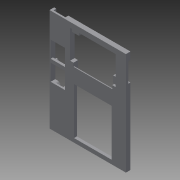
# Autodesk Inventor part: DisplayTop
Saved by Autodesk Inventor 2014 SP1 (Build 180222100, 222)
## iProperties
Created: 2014-03-24
Part Number: DisplayTop
Material: Generic
Document SubType Name: Modeling
Designer: patrigg
Density: 1 g/cm^3
Appearance: Default
Author: patrigg
Autodesk Inventor part; units mm, degrees
ref_plane "YZ Plane" through (0, 0, 0) normal (1, 0, 0) x (0, 1, 0)
ref_plane "XZ Plane" through (0, 0, 0) normal (0, 1, 0) x (-1, 0, 0)
ref_plane "XY Plane" through (0, 0, 0) normal (0, 0, 1) x (1, 0, 0)
sketch "Sketch2" plane through (0, 0, 0) normal (0, 1, 0) x (-1, 0, 0)
  line L0 (-33.5, -45) -> (33.5, -45)
  line L1 (33.5, -45) -> (33.5, 45)
  line L2 (33.5, 45) -> (-33.5, 45)
  line L3 (-33.5, 45) -> (-33.5, -45)
  line L4 (-33.5, -45) -> (33.5, 45) construction
  line L5 (33.5, -45) -> (-33.5, 45) construction
  point P0 (0, 0)
  dimension "d0" = 67
  dimension "d1" = 90
  constraints: 12 end point, 2 midpoint, 2 parallel, 1 horizontal, 1 perpendicular
  measures "d0" distance of L2.end L1.end
  measures "d1" distance of L1.end L0.end
extrude "Extrusion1" add sketch "Sketch2" along normal blind 4
sketch "Sketch3" plane through (0, 4, 0) normal (0, 1, 0) x (1, 0, 0)
  line L0 (33.5, 45) -> (-33.5, 45) projected
  line L1 (-14.5, -9.5) -> (23.5, -9.5)
  line L2 (23.5, -9.5) -> (23.5, 43)
  line L3 (23.5, 43) -> (-14.5, 43)
  line L4 (-14.5, 43) -> (-14.5, -9.5)
  line L5 (-14.5, -9.5) -> (23.5, 43) construction
  line L6 (23.5, -9.5) -> (-14.5, 43) construction
  line L7 (33.5, -45) -> (33.5, 45) projected
  point P0 (0, 0)
  point P1 (4.5, 16.75)
  dimension "d4" = 38
  dimension "d5" = 52.5
  dimension "d6" = 2
  dimension "d99" = 10
  constraints: 12 end point, 2 midpoint, 2 parallel, 1 horizontal, 1 perpendicular
  measures "d4" distance of L3.end L2.end
  measures "d5" distance of L2.end L1.end
  measures "d6" distance between parallel lines of L0 L3
  measures "d99" distance between parallel lines of L7 L2
extrude "Extrusion2" cut sketch "Sketch3" against normal blind 1.5
sketch "Sketch4" plane through (0, 2.5, 0) normal (0, 1, 0) x (1, 0, 0)
  line L0 (23.5, -9.5) -> (-14.5, -9.5) projected
  line L1 (23.5, 43) -> (23.5, -9.5) projected
  line L2 (-14.5, 43) -> (23.5, 43) projected
  line L3 (-14.5, -9.5) -> (-14.5, 43) projected
  line L4 (-12, 41.5) -> (21, 41.5)
  line L5 (21, 41.5) -> (21, 0.5)
  line L6 (21, 0.5) -> (-12, 0.5)
  line L7 (-12, 0.5) -> (-12, 41.5)
  line L8 (-12, 41.5) -> (21, 0.5) construction
  line L9 (21, 41.5) -> (-12, 0.5) construction
  point P0 (0, 0)
  point P1 (4.5, 21)
  dimension "d9" = 10
  dimension "d10" = 1.5
  dimension "d11" = 2.5
  dimension "d12" = 2.5
  constraints: 12 end point, 2 midpoint, 2 parallel, 1 horizontal, 1 perpendicular
  measures "d9" distance between parallel lines of L0 L6
  measures "d10" distance between parallel lines of L2 L4
  measures "d11" distance between parallel lines of L1 L5
  measures "d12" distance between parallel lines of L3 L7
extrude "Extrusion3" cut sketch "Sketch4" against normal blind 2.5 contours L4 L5 L6 L7
sketch "Sketch5" plane through (0, 4, 0) normal (0, 1, 0) x (1, 0, 0)
  line L0 (23.5, 43) -> (23.5, -9.5) projected
  line L1 (23.5, -9.5) -> (-14.5, -9.5) projected
  line L2 (-14.5, -9.5) -> (-14.5, 43) projected
  line L3 (-12.5, -15.5) -> (-12.5, -9.5)
  line L4 (21.5, -15.5) -> (21.5, -9.5)
  line L5 (33.5, 45) -> (-33.5, 45) projected
  line L6 (-12.5, -15.5) -> (21.5, -15.5)
  point P0 (0, 0)
  dimension "d18" = 2
  dimension "d19" = 2
  constraints: 6 end point, 2 perpendicular, 2 point on line, 1 parallel
  measures "d18" distance between parallel lines of L3 L2
  measures "d19" distance between parallel lines of L0 L4
extrude "Extrusion4" cut sketch "Sketch5" against normal blind 0.25
sketch "Sketch12" plane through (0, 4, 0) normal (0, 1, 0) x (1, 0, 0)
  line L0 (21.5, -15.5) -> (-12.5, -15.5) projected
  line L1 (-15.5, -40.5) -> (24.5, -40.5)
  line L2 (24.5, -40.5) -> (24.5, -15.5)
  line L3 (24.5, -15.5) -> (-15.5, -15.5)
  line L4 (-15.5, -15.5) -> (-15.5, -40.5)
  line L5 (-15.5, -40.5) -> (24.5, -15.5) construction
  line L6 (24.5, -40.5) -> (-15.5, -15.5) construction
  line L7 (23.5, 43) -> (23.5, -9.5) projected
  point P0 (0, 0)
  point P1 (4.5, -28)
  point P2 (4.5, -28)
  dimension "d58" = 40
  dimension "d59" = 25
  dimension "d100" = 1
  constraints: 12 end point, 3 midpoint, 2 parallel, 1 collinear, 1 horizontal, 1 perpendicular
  measures "d58" distance of L3.end L2.end
  measures "d59" distance of L2.end L1.end
  measures "d100" distance between parallel lines of L2 L7
extrude "Extrusion10" cut sketch "Sketch12" against normal blind 4
sketch "Sketch13" plane through (24.5, 4, 15.5) normal (-1, 0, 0) x (0, 0, 1)
  line L0 (0, 0) -> (25, 0) projected
  line L1 (0, 0) -> (0, -4) projected
  line L2 (25, -4) -> (0, -4) projected
  line L3 (6, 0) -> (6, -4)
  line L4 (0, -2.2) -> (6, -2.2)
  point P0 (-15.5, -4)
  dimension "d67" = 6
  dimension "d74" = 1.8
  constraints: 4 end point, 4 point on line, 2 perpendicular
  measures "d67" distance between parallel lines of L3 L1
  measures "d74" distance between parallel lines of L2 L4
sketch "Sketch14" plane through (-15.5, 4, 40.5) normal (1, 0, 0) x (0, 0, -1)
  line L0 (0, 0) -> (25, 0) projected
  line L1 (0, 0) -> (0, -4)
  line L2 (4.0418, -2.2) -> (4.0418, 0)
  line L3 (25, -4) -> (0, -4) projected
  line L4 (0, -2.2) -> (4.0418, -2.2)
  point P0 (40.5, -4)
  point P1 (0, -2)
  dimension "d79" = 1.8
  constraints: 6 end point, 2 perpendicular, 2 point on line, 1 midpoint
  measures "d79" distance between parallel lines of L3 L4
extrude "Extrusion13" add sketch "Sketch13" along normal blind 4 contours L0 L3 L4 L1
extrude "Extrusion14" add sketch "Sketch14" along normal blind 6
sketch "Sketch16" plane through (0, 3.75, 0) normal (0, 1, 0) x (1, 0, 0)
  line L0 (-12.5, -15.5) -> (-12.5, -9.5) projected
  line L1 (20.5, -15.5) -> (-12.5, -15.5) projected
  line L2 (21.5, -15.5) -> (20.5, -15.5) projected
  line L3 (21.5, -9.5) -> (21.5, -15.5) projected
  line L4 (-12.5, -9.5) -> (21.5, -9.5) projected
  point P0 (0, 0)
extrude "Extrusion15" cut sketch "Sketch16" against normal up to next
sketch "Sketch17" plane through (21.5, 4, 9.5) normal (-1, 0, 0) x (0, 0, 1)
  line L0 (0, -1.5) -> (0, -4) projected
  line L1 (6, -4) -> (0, -4) projected
  line L2 (6, -2.2) -> (6, -4) projected
  line L3 (6, 0) -> (6, -2.2) projected
  line L4 (0, -1.5) -> (-1.7339, -1.5) construction
  line L5 (5, -4) -> (7.1842, -4) construction
  line L6 (0, -1.5) -> (5, -4) construction
  arc A0 (2.5, -2.75) -> (0, -1.5) centre (0, -4.625) ccw
  line L7 (0, -1.5) -> (0, 0) projected
  line L8 (2.5, -2.75) -> (3.4375, -4)
  line L9 (2.9125, -4) -> (2.9125, -3.3)
  point P0 (-9.5, -4)
  dimension "d82" = 1
  dimension "d86" = 0.7
  constraints: 10 end point, 4 point on line, 2 parallel, 2 point on circle, 2 tangent, 1 centre point, 1 midpoint, 1 perpendicular
  measures "d82" distance from line of L2 L5.start
  measures "d86" distance of L9.start L9.end
extrude "Extrusion16" add sketch "Sketch17" along normal up to next contours A0 L8 L9 L1 L0
fillet "Fillet5" radius 1 1 edges at (4.5, 0.7, 12.4125)
sketch "Sketch18" plane through (0, 4, 0) normal (0, 1, 0) x (1, 0, 0)
  line L0 (-33.5, 45) -> (-33.5, -45) projected
  line L1 (-32.5, 9) -> (-20, 9)
  line L2 (-20, 9) -> (-20, -23)
  line L3 (-20, -23) -> (-32.5, -23)
  line L4 (-32.5, -23) -> (-32.5, 9)
  line L5 (33.5, 45) -> (-33.5, 45) projected
  point P0 (0, 0)
  dimension "d89" = 1
  dimension "d97" = 12.5
  dimension "d98" = 32
  dimension "d157" = 36
  constraints: 8 end point, 2 parallel, 1 horizontal, 1 perpendicular
  measures "d89" distance between parallel lines of L0 L4
  measures "d97" distance between parallel lines of L2 L4
  measures "d98" distance between parallel lines of L1 L3
  measures "d157" distance between parallel lines of L1 L5
extrude "Extrusion17" cut sketch "Sketch18" against normal up to next
sketch "Sketch19" plane through (-32.5, 4, 23) normal (1, 0, 0) x (0, 0, -1)
  line L0 (32, -4) -> (0, -4) projected
  line L1 (0, 0) -> (0, -4) projected
  line L2 (14.5, -4) -> (17.5, -4)
  line L3 (17.5, -4) -> (17.5, -2)
  line L4 (17.5, -2) -> (14.5, -2)
  line L5 (14.5, -2) -> (14.5, -4)
  line L6 (14.5, -4) -> (17.5, -2) construction
  line L7 (17.5, -4) -> (14.5, -2) construction
  point P0 (16, -3)
  dimension "d106" = 3
  dimension "d107" = 2
  dimension "d108" = 16
  constraints: 12 end point, 2 midpoint, 2 parallel, 1 collinear, 1 horizontal, 1 perpendicular
  measures "d106" distance of L4.end L3.end
  measures "d107" distance of L3.end L2.end
  measures "d108" distance from line of L1 point (16, -3)
extrude "Extrusion18" add sketch "Sketch19" along normal up to next
sketch "Sketch21" plane through (-32.5, 2, 8.5) normal (0, 1, 0) x (1, 0, 0)
  line L0 (0, 3) -> (12.5, 3) projected
  line L1 (0, 0) -> (12.5, 0) projected
  line L2 (4.75, 1) -> (7.75, 1)
  line L3 (7.75, 1) -> (7.75, 3)
  line L4 (7.75, 3) -> (4.75, 3)
  line L5 (4.75, 3) -> (4.75, 1)
  line L6 (4.75, 1) -> (7.75, 3) construction
  line L7 (7.75, 1) -> (4.75, 3) construction
  point P0 (32.5, 8.5)
  point P1 (6.25, 2)
  point P2 (6.25, 2)
  point P3 (6.25, 0)
  dimension "d111" = 3
  dimension "d112" = 2
  constraints: 12 end point, 4 midpoint, 2 parallel, 1 collinear, 1 horizontal, 1 perpendicular, 1 vertical alignment
  measures "d111" distance of L4.end L3.end
  measures "d112" distance of L3.end L2.end
extrude "Extrusion19" cut sketch "Sketch21" against normal blind 0.5
fillet "Fillet6" radius 1 1 edges at (-26.25, 1.5, 5.5)
sketch "Sketch22" plane through (-32.5, 2, 8.5) normal (0, 1, 0) x (1, 0, 0)
  line L0 (0, 0) -> (12.5, 0) projected
  line L1 (12.5, 3) -> (12.5, 0) projected
  circle A0 centre (2.125, 1.5) radius 1.25
  circle A1 centre (10.375, 1.5) radius 1.25
  point P0 (32.5, 8.5)
  point P1 (6.25, 1.5)
  point P2 (6.25, 0)
  point P3 (12.5, 1.5)
  dimension "d116" = 2.5
  dimension "d117" = 2.5
  dimension "d118" = 8.25
  dimension "d119" = 4.125
  constraints: 3 horizontal alignment, 2 centre point, 2 midpoint, 1 vertical alignment
  measures "d116" diameter of A0
  measures "d117" diameter of A1
  measures "d118" distance of A1.centre A0.centre
  measures "d119" distance of A0.centre point (6.25, 1.5)
extrude "Extrusion20" add sketch "Sketch22" along normal blind 2
chamfer "Chamfer3" distance 0.5 angle 45 2 edges at (-31.625, 4, 7) (-23.375, 4, 7)
sketch "Sketch23" plane through (0, 4, 0) normal (0, 1, 0) x (1, 0, 0)
  line L0 (-33.5, 45) -> (-33.5, -45) projected
  line L1 (-33.5, -45) -> (33.5, -45) projected
  line L2 (-31.5, -29) -> (-21, -29)
  line L3 (-21, -29) -> (-21, -45)
  line L4 (-21, -45) -> (-31.5, -45)
  line L5 (-31.5, -45) -> (-31.5, -29)
  line L6 (-31.5, -29) -> (-21, -45) construction
  line L7 (-21, -29) -> (-31.5, -45) construction
  line L8 (21.5, -9.5) -> (21.5, -15.5) projected
  line L9 (-31.25, -29) -> (-31.25, -37)
  line L10 (-31.25, -37) -> (-31.5, -37)
  line L11 (-21.25, -29) -> (-21.25, -37)
  line L12 (-21.25, -37) -> (-21, -37)
  point P0 (0, 0)
  point P1 (-26.25, -37)
  dimension "d125" = 10.5
  dimension "d126" = 16
  dimension "d127" = 7.25
  dimension "d130" = 0.25
  dimension "d131" = 0.25
  dimension "d132" = 8
  constraints: 20 end point, 4 midpoint, 4 perpendicular, 3 parallel, 2 collinear, 2 point on line, 1 horizontal
  measures "d125" distance of L3.end L4.end
  measures "d126" distance of L2.end L3.end
  measures "d127" distance from line of L0 point (-26.25, -37)
  measures "d130" distance between parallel lines of L5 L9
  measures "d131" distance between parallel lines of L3 L11
  measures "d132" distance of L4.end L10.end
extrude "Extrusion22" cut sketch "Sketch23" against normal blind 2.5 contours L5 L10 L9 L2 L11 L12 L3 L1
sketch "Sketch24" plane through (0, 4, 0) normal (0, 1, 0) x (1, 0, 0)
  line L0 (21.5, -15.5) -> (20.5, -15.5) projected
  line L1 (-31.25, -37) -> (-31.25, -29) projected
  line L2 (-31.25, -29) -> (-21.25, -29) projected
  line L3 (-21.25, -29) -> (-21.25, -37) projected
  line L4 (-32.5, 9) -> (-20, 9) projected
  line L5 (-20, 9) -> (-20, -23) projected
  line L6 (-20, -23) -> (-32.5, -23) projected
  line L7 (-27.5, 9) -> (-27.5, 17.5)
  line L8 (-27.5, 17.5) -> (-16.5, 17.5)
  line L9 (-16.5, 17.5) -> (-16.5, -29)
  line L10 (-16.5, -29) -> (-21.25, -29)
  line L11 (-25, 9) -> (-25, 15)
  line L12 (-25, 15) -> (-19, 15)
  line L13 (-19, 15) -> (-19, -25)
  line L14 (-19, -25) -> (-28.25, -25)
  line L15 (-28.25, -25) -> (-28.25, -29)
  point P0 (0, 0)
  point P1 (-26.25, 9)
  point P2 (-26.25, 9)
  dimension "d135" = 2.5
  dimension "d136" = 2.5
  dimension "d137" = 2.5
  dimension "d138" = 4
  dimension "d139" = 1
  dimension "d140" = 6
  dimension "d141" = 3
  dimension "d142" = 1.25
  constraints: 18 end point, 7 perpendicular, 3 parallel, 3 point on line, 2 midpoint, 1 coincident
  measures "d135" distance between parallel lines of L11 L7
  measures "d136" distance between parallel lines of L8 L12
  measures "d137" distance between parallel lines of L9 L13
  measures "d138" distance between parallel lines of L10 L14
  measures "d139" distance between parallel lines of L5 L13
  measures "d140" distance between parallel lines of L4 L12
  measures "d141" distance between parallel lines of L15 L1
  measures "d142" distance from line of L7 point (-26.25, 9)
extrude "Extrusion23" cut sketch "Sketch24" against normal blind 2.5
fillet "Fillet7" radius 2 8 edges at (-25, 2.75, -15) (-19, 2.75, -15) (-19, 2.75, 25) (-16.5, 2.75, 29) (-28.25, 2.75, 25) (-21.25, 2.75, 29) (-16.5, 2.75, -17.5) (-27.5, 2.75, -17.5)
chamfer "Chamfer4" distance 2 angle 45 2 edges at (-27.5, 2.75, -9) (-25, 2.75, -9)
fillet "Fillet8" radius 2 4 edges at (-29.5, 2.75, -9) (-27.5, 2.75, -11) (-25, 2.75, -11) (-23, 2.75, -9)
sketch "Sketch25" plane through (0, 4, 0) normal (0, 1, 0) x (1, 0, 0)
  line L0 (33.5, -45) -> (33.5, 45) projected
  line L1 (24.5, -21.5) -> (24.5, -40.5) projected
  line L2 (24.5, -40.5) -> (-9.5, -40.5) projected
  line L3 (24.5, -21.5) -> (33.5, -21.5)
  line L4 (24.5, -38.5) -> (33.5, -38.5)
  point P0 (0, 0)
  dimension "d150" = 2
  constraints: 4 end point, 3 point on line, 1 parallel, 1 perpendicular
  measures "d150" distance between parallel lines of L2 L4
extrude "Extrusion24" cut sketch "Sketch25" against normal blind 2
body "Solid1"
